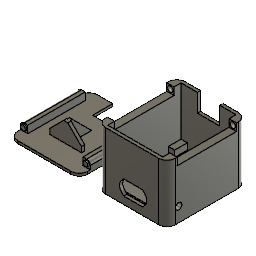
WirelessTéléInfo v8 (Autodesk Fusion 360 design; units mm, degrees)
Autodesk Fusion 360 part; units mm, degrees
form "Form1" [no effect]
sketch "Bases" plane through (0, 0, 0) normal (0, 1, 0) x (1, 0, 0)
  line L0 (7.8348, 4.1595) -> (32.8348, 4.1595)
  line L1 (36.8348, 8.1595) -> (36.8348, 37.7595)
  line L2 (32.8348, 41.7595) -> (7.8348, 41.7595)
  line L3 (3.8348, 37.7595) -> (3.8348, 8.1595)
  arc A0 (7.8348, 41.7595) -> (3.8348, 37.7595) centre (7.8348, 37.7595) ccw
  arc A1 (36.8348, 37.7595) -> (32.8348, 41.7595) centre (32.8348, 37.7595) ccw
  arc A2 (32.8348, 4.1595) -> (36.8348, 8.1595) centre (32.8348, 8.1595) ccw
  arc A3 (3.8348, 8.1595) -> (7.8348, 4.1595) centre (7.8348, 8.1595) ccw
  arc A4 (3.8348, 8.1595) -> (7.8348, 4.1595) centre (7.8348, 8.1595) ccw
  arc A5 (32.8348, 4.1595) -> (36.8348, 8.1595) centre (32.8348, 8.1595) ccw
  line L4 (3.8348, 37.7595) -> (3.8348, 8.1595)
  line L5 (36.8348, 8.1595) -> (36.8348, 37.7595)
  line L6 (7.8348, 4.1595) -> (32.8348, 4.1595)
  arc A6 (7.8348, 41.7595) -> (3.8348, 37.7595) centre (7.8348, 37.7595) ccw
  line L7 (32.8348, 41.7595) -> (7.8348, 41.7595)
  arc A7 (36.8348, 37.7595) -> (32.8348, 41.7595) centre (32.8348, 37.7595) ccw
  line L8 (-37.5541, 37.6977) -> (-37.5541, 8.0977)
  arc A8 (-8.5541, 4.0977) -> (-4.5541, 8.0977) centre (-8.5541, 8.0977) ccw
  line L9 (-33.5541, 4.0977) -> (-8.5541, 4.0977)
  line L10 (-8.5541, 41.6977) -> (-33.5541, 41.6977)
  arc A9 (-33.5541, 41.6977) -> (-37.5541, 37.6977) centre (-33.5541, 37.6977) ccw
  arc A10 (-4.5541, 37.6977) -> (-8.5541, 41.6977) centre (-8.5541, 37.6977) ccw
  arc A11 (-37.5541, 8.0977) -> (-33.5541, 4.0977) centre (-33.5541, 8.0977) ccw
  line L11 (-4.5541, 8.0977) -> (-4.5541, 37.6977)
  line L12 (-37.5541, 36.4977) -> (-34.0541, 36.4977)
  line L13 (-34.0541, 36.4977) -> (-34.0541, 9.2977)
  line L14 (-34.0541, 9.2977) -> (-37.5541, 9.2977)
  line L15 (-37.5541, 9.2977) -> (-37.5541, 36.4977)
  line L16 (-4.5541, 36.4977) -> (-8.0541, 36.4977)
  line L17 (-8.0541, 36.4977) -> (-8.0541, 9.2977)
  line L18 (-8.0541, 9.2977) -> (-4.5541, 9.2977)
  line L19 (-4.5541, 9.2977) -> (-4.5541, 36.4977)
  dimension "d14" = 4
  dimension "d15" = 4
  dimension "d16" = 37.6
  dimension "d18" = 33
  dimension "d31" = 4
  dimension "d32" = 4
  dimension "d33" = 37.6
  dimension "d34" = 33
  dimension "d35" = 4
  dimension "d36" = 4
  dimension "d37" = 37.6
  dimension "d38" = 33
  dimension "d45" = 27.2
  dimension "d46" = 3.5
  dimension "d47" = 3.5
  measures "d14" radius of A0
  measures "d15" radius of A1
  measures "d16" distance of L0 L2
  measures "d18" distance of L1 L3
  measures "d31" radius of A6
  measures "d32" radius of A7
  measures "d33" distance of L6 L7
  measures "d34" distance of L4 L5
  measures "d35" radius of A9
  measures "d36" radius of A10
  measures "d37" distance of L9 L10
  measures "d38" distance of L8 L11
  measures "d45" distance of origin
extrude "Extrude1" add sketch "Bases" along normal blind 27.25 contours L0 L1 L2 L3 A0 A1 A2 A3 A4 A5 L4 L5 L6 A6 L7 A7 makes body 1
sketch "TopBox" plane through (0, 27.25, 0) normal (0, 1, 0) x (-1, 0, 0)
  arc A0 (-3.8348, -8.1595) -> (-7.8348, -4.1595) centre (-7.8348, -8.1595) ccw
  line L0 (-7.8348, -4.1595) -> (-32.8348, -4.1595)
  arc A1 (-32.8348, -4.1595) -> (-36.8348, -8.1595) centre (-32.8348, -8.1595) ccw
  line L1 (-36.8348, -8.1595) -> (-36.8348, -37.7595)
  arc A2 (-36.8348, -37.7595) -> (-32.8348, -41.7595) centre (-32.8348, -37.7595) ccw
  line L2 (-32.8348, -41.7595) -> (-7.8348, -41.7595)
  arc A3 (-7.8348, -41.7595) -> (-3.8348, -37.7595) centre (-7.8348, -37.7595) ccw
  line L3 (-3.8348, -37.7595) -> (-3.8348, -8.1595)
  line L4 (-7.3348, -5.6595) -> (-33.3348, -5.6595)
  line L5 (-33.3348, -5.6595) -> (-33.3348, -40.2595)
  line L6 (-33.3348, -40.2595) -> (-7.3348, -40.2595)
  line L7 (-7.3348, -40.2595) -> (-7.3348, -5.6595)
  line L8 (-3.8348, -36.9595) -> (-7.3348, -36.9595)
  line L9 (-7.3348, -36.9595) -> (-7.3348, -8.9595)
  line L10 (-7.3348, -8.9595) -> (-3.8348, -8.9595)
  line L11 (-3.8348, -8.9595) -> (-3.8348, -36.9595)
  line L12 (-33.3348, -36.9595) -> (-36.8348, -36.9595)
  line L13 (-36.8348, -36.9595) -> (-36.8348, -8.9595)
  line L14 (-36.8348, -8.9595) -> (-33.3348, -8.9595)
  line L15 (-33.3348, -8.9595) -> (-33.3348, -36.9595)
  dimension "d22" = 34.6
  dimension "d23" = 26
  dimension "d24" = 1.5
  dimension "d25" = 3.5
  dimension "d28" = 28
  measures "d24" distance of L0 L4
  measures "d25" distance of L3 L7
extrude "Extrude2" cut sketch "TopBox" against normal blind 26 contours L4 L5 L6 L7 L9 L15 bodies 1
extrude "Extrude3" cut sketch "TopBox" against normal blind 3.5 contours L3 L7 L8 L9 L10 L11 | L1 L5 L12 L13 L14 L15 bodies 1
extrude "Extrude4" add sketch "Bases" along normal blind 1.25 separate body contours L8 A8 L9 L10 A9 A10 A11 L11 L12 L13 L14 L16 L17 L18 | L8 L12 L13 L14 L15 | L11 L16 L17 L18 L19 makes body 2
extrude "Extrude5" add sketch "Bases" along normal blind 4.75 contours L8 L12 L13 L14 L15 | L11 L16 L17 L18 L19 bodies 2
fillet "Fillet1" radius 1.75 1 edges at (-4.5541, 4.75, -22.8977) on bodies 2
fillet "Fillet1" radius 1.75 1 edges at (-37.5541, 4.75, -22.8977) on bodies 2
sphere "SpherePrimitive8" cut diameter 2.5 placed x (1, 0, 0) y (0, 1, 0) z (0, 0, 1) at (35.0848, 25.5, -36.9595) bodies 1
pattern_linear "R-Pattern1" count 2 spacing 28 along (0, 0, 1) count 2 spacing 29.5 along (-1, 0, 0) of "SpherePrimitive8"
sphere "SpherePrimitive9" add diameter 2.5 placed x (-1, 0, 0) y (0, 1, 0) z (0, 0, -1) at (-6.3041, 3, -36.4977) bodies 2
pattern_linear "R-Pattern2" count 2 spacing 27.2 along (0, 0, 1) count 2 spacing 29.5 along (-1, 0, 0) of "SpherePrimitive9"
sketch "CutSpheres" plane through (0, 1.25, 0) normal (0, 1, 0) x (-1, 0, 0)
  line L0 (8.0541, -36.4977) -> (4.5541, -36.4977)
  line L1 (4.5541, -36.4977) -> (4.5541, -37.6977)
  arc A0 (4.5541, -37.6977) -> (8.5541, -41.6977) centre (8.5541, -37.6977) ccw
  line L2 (8.5541, -41.6977) -> (33.5541, -41.6977)
  arc A1 (33.5541, -41.6977) -> (37.5541, -37.6977) centre (33.5541, -37.6977) ccw
  line L3 (37.5541, -37.6977) -> (37.5541, -36.4977)
  line L4 (37.5541, -36.4977) -> (34.0541, -36.4977)
  line L5 (34.0541, -36.4977) -> (34.0541, -9.2977)
  line L6 (34.0541, -9.2977) -> (37.5541, -9.2977)
  line L7 (37.5541, -9.2977) -> (37.5541, -8.0977)
  arc A2 (37.5541, -8.0977) -> (33.5541, -4.0977) centre (33.5541, -8.0977) ccw
  line L8 (33.5541, -4.0977) -> (8.5541, -4.0977)
  arc A3 (8.5541, -4.0977) -> (4.5541, -8.0977) centre (8.5541, -8.0977) ccw
  line L9 (4.5541, -8.0977) -> (4.5541, -9.2977)
  line L10 (4.5541, -9.2977) -> (8.0541, -9.2977)
  line L11 (8.0541, -9.2977) -> (8.0541, -36.4977)
  line L12 (7.5541, -37.7477) -> (5.0541, -37.7477)
  line L13 (5.0541, -37.7477) -> (5.0541, -37.0477)
  line L14 (5.0541, -37.0477) -> (7.5541, -37.0477)
  line L15 (7.5541, -37.0477) -> (7.5541, -37.7477)
  line L16 (4.5541, -8.0977) -> (4.5541, -37.6977)
  line L17 (4.5541, -36.4977) -> (8.0541, -36.4977)
  line L18 (7.5541, -8.7477) -> (5.0541, -8.7477)
  line L19 (5.0541, -8.7477) -> (5.0541, -8.0477)
  line L20 (5.0541, -8.0477) -> (7.5541, -8.0477)
  line L21 (7.5541, -8.0477) -> (7.5541, -8.7477)
  line L22 (37.0541, -8.7477) -> (34.5541, -8.7477)
  line L23 (34.5541, -8.7477) -> (34.5541, -8.0477)
  line L24 (34.5541, -8.0477) -> (37.0541, -8.0477)
  line L25 (37.0541, -8.0477) -> (37.0541, -8.7477)
  line L26 (37.0541, -37.7477) -> (34.5541, -37.7477)
  line L27 (34.5541, -37.7477) -> (34.5541, -37.0477)
  line L28 (34.5541, -37.0477) -> (37.0541, -37.0477)
  line L29 (37.0541, -37.0477) -> (37.0541, -37.7477)
  line L30 (8.0541, -9.2977) -> (4.5541, -9.2977)
  line L31 (34.0541, -9.2977) -> (37.5541, -9.2977)
  line L32 (37.5541, -36.4977) -> (34.0541, -36.4977)
  line L33 (37.5541, -37.6977) -> (37.5541, -8.0977)
  dimension "d71" = 0.5
  dimension "d72" = 2.5
  dimension "d73" = 0.55
  dimension "d74" = 0.7
  dimension "d77" = 0.55
  dimension "d78" = 0.55
  dimension "d79" = 0.55
  dimension "d80" = 0.7
  dimension "d81" = 0.7
  dimension "d82" = 0.7
  dimension "d83" = 0.5
  dimension "d84" = 0.5
  dimension "d85" = 0.5
  dimension "d86" = 2.5
  dimension "d87" = 2.5
  dimension "d88" = 2.5
  measures "d71" distance of L13 L16
  measures "d73" distance of L14 L17
  measures "d77" distance of L18 L30
  measures "d78" distance of L22 L31
  measures "d79" distance of L28 L32
  measures "d83" distance of L16 L19
  measures "d84" distance of L25 L33
  measures "d85" distance of L29 L33
extrude "Extrude6" cut sketch "CutSpheres" along normal blind 3 contours L12 L13 L14 L15 | L18 L19 L20 L21 | L22 L23 L24 L25 | L26 L27 L28 L29 bodies 2
sketch "Supports" plane through (0, 1.25, 0) normal (0, 1, 0) x (-1, 0, 0)
  line L0 (-7.3348, -40.2595) -> (-7.3348, -5.6595)
  line L1 (-7.3348, -5.6595) -> (-33.3348, -5.6595)
  line L2 (-33.3348, -5.6595) -> (-33.3348, -40.2595)
  line L3 (-33.3348, -40.2595) -> (-7.3348, -40.2595)
  line L4 (-7.3348, -5.6595) -> (-29.3348, -5.6595)
  line L5 (-29.3348, -5.6595) -> (-29.3348, -11.6595)
  line L6 (-29.3348, -11.6595) -> (-7.3348, -11.6595)
  line L7 (-7.3348, -11.6595) -> (-7.3348, -5.6595)
  line L8 (-7.3348, -40.2595) -> (-10.3348, -40.2595)
  line L9 (-10.3348, -40.2595) -> (-10.3348, -34.2595)
  line L10 (-10.3348, -34.2595) -> (-7.3348, -34.2595)
  line L11 (-7.3348, -34.2595) -> (-7.3348, -40.2595)
  line L12 (-33.3348, -40.2595) -> (-30.3348, -40.2595)
  line L13 (-30.3348, -40.2595) -> (-30.3348, -34.2595)
  line L14 (-30.3348, -34.2595) -> (-33.3348, -34.2595)
  line L15 (-33.3348, -34.2595) -> (-33.3348, -40.2595)
  dimension "d93" = 6
  dimension "d94" = 22
  dimension "d95" = 6
  dimension "d96" = 6
  dimension "d97" = 3
  dimension "d98" = 3
extrude "Extrude7" add sketch "Supports" along normal blind 3 contours L0 L3 L8 L9 L10 L11 | L0 L1 L4 L5 L6 L7 | L2 L3 L12 L13 L14 L15 bodies 1
sketch "ResetHole" plane through (36.8348, 0, 0) normal (1, 0, 0) x (0, 0, -1)
  line L0 (8.9595, 23.75) -> (8.9595, 27.25)
  line L1 (8.1595, 27.25) -> (8.1595, 0)
  line L2 (8.1595, 0) -> (37.7595, 0)
  line L3 (37.7595, 0) -> (37.7595, 27.25)
  line L4 (36.9595, 27.25) -> (36.9595, 23.75)
  line L5 (36.9595, 23.75) -> (8.9595, 23.75)
  circle A0 centre (9.6595, 6.85) radius 1.5
  line L6 (8.1595, 0) -> (37.7595, 0)
  line L7 (8.9595, 27.25) -> (8.1595, 27.25)
  line L8 (37.7595, 27.25) -> (36.9595, 27.25)
  dimension "d101" = 1.5
  dimension "d102" = 3
  dimension "d103" = 6.85
  measures "d101" distance of L1
  measures "d102" diameter of A0
  measures "d103" distance of L6
extrude "Extrude8" cut sketch "ResetHole" against normal blind 3.5 contours A0 bodies 1
sketch "USBHole" plane through (0, 0, -4.1595) normal (0, 0, 1) x (1, 0, 0)
  line L0 (7.8348, 0) -> (32.8348, 0)
  line L1 (32.8348, 0) -> (32.8348, 27.25)
  line L2 (32.8348, 27.25) -> (7.8348, 27.25)
  line L3 (7.8348, 27.25) -> (7.8348, 0)
  line L4 (16.3348, 10.55) -> (25.3348, 10.55)
  line L5 (25.3348, 3.55) -> (16.3348, 3.55)
  spline S0 degree 5 poles (16.3348, 10.55) (16.188, 10.41) (15.907, 10.13) (15.5241, 9.71) (15.0918, 9.15) (14.6906, 8.45) (14.4412, 7.75) (14.3558, 7.05) (14.4412, 6.35) (14.6906, 5.65) (15.0918, 4.95) (15.5241, 4.39) (15.907, 3.97) (16.188, 3.69) (16.3348, 3.55) knots 0 0 0 0 0 0 0.1 0.2 0.3 0.4 0.5 0.6 0.7 0.8 0.9 1 1 1 1 1 1
  spline S1 degree 5 poles (25.3348, 3.55) (25.4817, 3.69) (25.7626, 3.97) (26.1456, 4.39) (26.5779, 4.95) (26.979, 5.65) (27.2285, 6.35) (27.3139, 7.05) (27.2285, 7.75) (26.979, 8.45) (26.5779, 9.15) (26.1456, 9.71) (25.7626, 10.13) (25.4817, 10.41) (25.3348, 10.55) knots 0 0 0 0 0 0 0.1 0.2 0.3 0.4 0.5 0.6 0.7 0.8 0.9 1 1 1 1 1 1
  line L6 (16.3348, 10.55) -> (16.3348, 3.55)
  line L7 (25.3348, 10.55) -> (25.3348, 3.55)
  line L8 (7.8348, 3.55) -> (32.8348, 3.55)
  line L9 (7.8348, 0) -> (32.8348, 0)
  dimension "d104" = 9
  dimension "d105" = 7
  dimension "d106" = 4
  dimension "d107" = 4
  dimension "d108" = 4
  dimension "d109" = 4
  dimension "d115" = 7.05
  dimension "d138" = 4
  measures "d115" distance of L9
extrude "Extrude9" cut sketch "USBHole" against normal blind 1.5 contours L4 L5 L6 L7 L8 | S0 L6 | S1 L7 bodies 1
sketch "BornierHole" plane through (0, 0, -41.7595) normal (0, 0, -1) x (-1, 0, 0)
  line L0 (-32.8348, 0) -> (-7.8348, 0)
  line L1 (-7.8348, 0) -> (-7.8348, 27.25)
  line L2 (-7.8348, 27.25) -> (-32.8348, 27.25)
  line L3 (-32.8348, 27.25) -> (-32.8348, 0)
  line L4 (-25.5848, 27.25) -> (-15.0848, 27.25)
  line L5 (-15.0848, 27.25) -> (-15.0848, 18.75)
  line L6 (-15.0848, 18.75) -> (-25.5848, 18.75)
  line L7 (-25.5848, 18.75) -> (-25.5848, 27.25)
  dimension "d116" = 10.5
  dimension "d117" = 8.5
  measures "d116" distance of origin
  measures "d117" distance of origin
extrude "Extrude10" cut sketch "BornierHole" against normal blind 1.5 contours L2 L4 L5 L6 L7 bodies 1
sketch "BordnierHoleAndMaintainLeg" plane through (0, 1.25, 0) normal (0, 1, 0) x (-1, 0, 0)
  line L0 (8.0541, -36.4977) -> (4.5541, -36.4977)
  line L1 (4.5541, -36.4977) -> (4.5541, -37.6977)
  arc A0 (4.5541, -37.6977) -> (8.5541, -41.6977) centre (8.5541, -37.6977) ccw
  line L2 (8.5541, -41.6977) -> (33.5541, -41.6977)
  arc A1 (33.5541, -41.6977) -> (37.5541, -37.6977) centre (33.5541, -37.6977) ccw
  line L3 (37.5541, -37.6977) -> (37.5541, -36.4977)
  line L4 (37.5541, -36.4977) -> (34.0541, -36.4977)
  line L5 (34.0541, -36.4977) -> (34.0541, -9.2977)
  line L6 (34.0541, -9.2977) -> (37.5541, -9.2977)
  line L7 (37.5541, -9.2977) -> (37.5541, -8.0977)
  arc A2 (37.5541, -8.0977) -> (33.5541, -4.0977) centre (33.5541, -8.0977) ccw
  line L8 (33.5541, -4.0977) -> (8.5541, -4.0977)
  arc A3 (8.5541, -4.0977) -> (4.5541, -8.0977) centre (8.5541, -8.0977) ccw
  line L9 (4.5541, -8.0977) -> (4.5541, -9.2977)
  line L10 (4.5541, -9.2977) -> (8.0541, -9.2977)
  line L11 (8.0541, -9.2977) -> (8.0541, -36.4977)
  line L12 (26.3041, -41.6977) -> (15.8041, -41.6977)
  line L13 (15.8041, -41.6977) -> (15.8041, -32.1977)
  line L14 (15.8041, -32.1977) -> (26.3041, -32.1977)
  line L15 (26.3041, -32.1977) -> (26.3041, -41.6977)
  line L16 (28.5541, -14.1977) -> (13.5541, -14.1977)
  line L17 (13.5541, -14.1977) -> (13.5541, -15.6977)
  line L18 (13.5541, -15.6977) -> (28.5541, -15.6977)
  line L19 (28.5541, -15.6977) -> (28.5541, -14.1977)
  line L20 (21.8041, -15.6977) -> (20.3041, -15.6977)
  line L21 (20.3041, -15.6977) -> (20.3041, -25.6977)
  line L22 (20.3041, -25.6977) -> (21.8041, -25.6977)
  line L23 (21.8041, -25.6977) -> (21.8041, -15.6977)
  line L24 (34.0541, -14.1977) -> (8.0541, -14.1977)
  dimension "d120" = 10.5
  dimension "d121" = 9.5
  dimension "d122" = 1.5
  dimension "d123" = 1.5
  dimension "d124" = 15
  dimension "d125" = 10
  dimension "d126" = 27.5
  measures "d120" distance of origin
  measures "d122" distance of L16 L18
  measures "d123" distance of L21 L23
  measures "d125" distance of origin
  measures "d126" distance of L2 L24
extrude "Extrude11" cut sketch "BordnierHoleAndMaintainLeg" against normal blind 1.25 contours L2 L12 L13 L14 L15 bodies 2
extrude "Extrude12" add sketch "BordnierHoleAndMaintainLeg" along normal blind 9 contours L16 L17 L18 L19 L20 L24 | L18 L20 L21 L22 L23 bodies 2
chamfer "Chamfer1" distance 6.5 angle 45 2 edges at (-28.5541, 10.25, -14.9477) (-13.5541, 10.25, -14.9477) on bodies 2
chamfer "Chamfer2" distance 9 angle 45 1 edges at (-21.0541, 10.25, -25.6977) on bodies 2
sketch "ModuleName" plane through (0, 0, 0) normal (0, -1, 0) x (1, 0, 0)
  line L0 (-26.3041, -41.6977) -> (-26.3041, -32.1977)
  line L1 (-26.3041, -32.1977) -> (-15.8041, -32.1977)
  line L2 (-15.8041, -32.1977) -> (-15.8041, -41.6977)
  line L3 (-15.8041, -41.6977) -> (-8.5541, -41.6977)
  arc A0 (-8.5541, -41.6977) -> (-4.5541, -37.6977) centre (-8.5541, -37.6977) ccw
  line L4 (-4.5541, -37.6977) -> (-4.5541, -8.0977)
  arc A1 (-4.5541, -8.0977) -> (-8.5541, -4.0977) centre (-8.5541, -8.0977) ccw
  line L5 (-8.5541, -4.0977) -> (-33.5541, -4.0977)
  arc A2 (-33.5541, -4.0977) -> (-37.5541, -8.0977) centre (-33.5541, -8.0977) ccw
  line L6 (-37.5541, -8.0977) -> (-37.5541, -37.6977)
  arc A3 (-37.5541, -37.6977) -> (-33.5541, -41.6977) centre (-33.5541, -37.6977) ccw
  line L7 (-33.5541, -41.6977) -> (-26.3041, -41.6977)
  line L8 (-8.3337, -24.7187) -> (-33.0602, -24.7187) construction
  line L9 (-33.0602, -24.7187) -> (-33.0602, -29.7187) construction
  line L10 (-33.0602, -29.7187) -> (-8.3337, -29.7187) construction
  line L11 (-8.3337, -29.7187) -> (-8.3337, -24.7187) construction
  line L12 (-10.3438, -18.9177) -> (-30.6074, -18.9177) construction
  line L13 (-30.6074, -18.9177) -> (-30.6074, -23.9177) construction
  line L14 (-30.6074, -23.9177) -> (-10.3438, -23.9177) construction
  line L15 (-10.3438, -23.9177) -> (-10.3438, -18.9177) construction
  line L16 (-10.9219, -13.5277) -> (-29.8037, -13.5277) construction
  line L17 (-29.8037, -13.5277) -> (-29.8037, -18.5277) construction
  line L18 (-29.8037, -18.5277) -> (-10.9219, -18.5277) construction
  line L19 (-10.9219, -18.5277) -> (-10.9219, -13.5277) construction
  line L20 (-15.3778, -7.1463) -> (-24.8529, -7.1463) construction
  line L21 (-24.8529, -7.1463) -> (-24.8529, -12.1463) construction
  line L22 (-24.8529, -12.1463) -> (-15.3778, -12.1463) construction
  line L23 (-15.3778, -12.1463) -> (-15.3778, -7.1463) construction
  text T0 "DomoChip" font "Arial" height 5 bold align ink ink in box 0 x 0 at (-8.3337, -24.7187) x (-1, 0) y (0, -1) spacing 1 kerned height is em
  text T1 "Wireless" font "Arial" height 5 bold align ink ink in box 0 x 0 at (-10.3438, -18.9177) x (-1, 0) y (0, -1) spacing 1 kerned height is em
  text T2 "TéléInfo" font "Arial" height 5 bold align ink ink in box 0 x 0 at (-10.9219, -13.5277) x (-1, 0) y (0, -1) spacing 1 kerned height is em
  text T3 "V2.1" font "Arial" height 5 bold align ink ink in box 0 x 0 at (-15.3778, -7.1463) x (-1, 0) y (0, -1) spacing 1 kerned height is em
extrude "Extrude13" cut sketch "ModuleName" against normal blind 0.5 text T0 T1 T2 T3 bodies 2
equation "_width = 34.6 mm" comment "width of the box (affects the length of the hinges)"
equation "_length = 26 mm" comment "length of the box"
equation "_height = 26 mm" comment "height of the box"
equation "_rounding = 4 mm" comment "rounding radius of the corners of the box"
equation "_minimumWallThickness = 0.5 mm" comment "thickness of the walls around the magnets"
equation "_sidewallThickness = 1.5 mm" comment "thickness of the side walls without the hinge"
equation "_horizontalThickness = 1.25 mm" comment "thickness of the bottom of the box or the top of the lid"
equation "_magnetDiameter = 2.5 mm" comment "diameter of magnets in the hinge"
equation "_magnetHeight = 1 mm" comment "height magnets in the hinge"
equation "_hingeGap = 0.4 mm" comment "gap bewteen the lid and box parts"
equation "_hingeOverlap = 0.15 mm" comment "Size of lid's spheres that go into box holes"
equation "d14 = _rounding"
equation "d15 = _rounding"
equation "d16 = _width + 2 * _sidewallThickness"
equation "d18 = _length + 4 * _minimumWallThickness + 2 * _magnetDiameter"
equation "d20 = _height + _horizontalThickness"
equation "d22 = _width"
equation "d23 = _length"
equation "d24 = _sidewallThickness"
equation "d25 = 2 * _minimumWallThickness + _magnetDiameter"
equation "d26 = -_height"
equation "d28 = _width + 2 * _sidewallThickness - 2 * _rounding - 2 * _magnetHeight + _hingeGap"
equation "d29 = -_magnetDiameter - 2 * _minimumWallThickness"
equation "d31 = _rounding"
equation "d32 = _rounding"
equation "d33 = _width + 2 * _sidewallThickness"
equation "d34 = _length + 4 * _minimumWallThickness + 2 * _magnetDiameter"
equation "d35 = _rounding"
equation "d36 = _rounding"
equation "d37 = _width + 2 * _sidewallThickness"
equation "d38 = _length + 4 * _minimumWallThickness + 2 * _magnetDiameter"
equation "d43 = _horizontalThickness"
equation "d45 = _width + 2 * _sidewallThickness - 2 * _rounding - 2 * _magnetHeight - _hingeGap"
equation "d46 = _magnetDiameter + 2 * _minimumWallThickness"
equation "d47 = _magnetDiameter + 2 * _minimumWallThickness"
equation "d48 = _horizontalThickness + _magnetDiameter + 2 * _minimumWallThickness"
equation "d50 = ( _magnetDiameter + 2 * _minimumWallThickness ) / 2"
equation "d51 = ( _magnetDiameter + 2 * _minimumWallThickness ) / 2"
equation "d59 = _width + 2 * _sidewallThickness - 2 * _rounding - 2 * _magnetHeight + _hingeGap"
equation "d60 = -_length - _magnetDiameter - 2 * _minimumWallThickness"
equation "d64 = _width + 2 * _sidewallThickness - 2 * _rounding - 2 * _magnetHeight - _hingeGap"
equation "d65 = -_length - _magnetDiameter - 2 * _minimumWallThickness"
equation "d71 = _minimumWallThickness"
equation "d72 = _magnetDiameter"
equation "d73 = _hingeGap + _hingeOverlap"
equation "d74 = _magnetDiameter / 2 - _hingeGap - _hingeOverlap"
equation "d75 = _minimumWallThickness + _magnetDiameter"
equation "d77 = _hingeGap + _hingeOverlap"
equation "d78 = _hingeGap + _hingeOverlap"
equation "d79 = _hingeGap + _hingeOverlap"
equation "d80 = _magnetDiameter / 2 - _hingeGap - _hingeOverlap"
equation "d81 = _magnetDiameter / 2 - _hingeGap - _hingeOverlap"
equation "d82 = _magnetDiameter / 2 - _hingeGap - _hingeOverlap"
equation "d83 = _minimumWallThickness"
equation "d84 = _minimumWallThickness"
equation "d85 = _minimumWallThickness"
equation "d86 = _magnetDiameter"
equation "d87 = _magnetDiameter"
equation "d88 = _magnetDiameter"
equation "d101 = 4 mm - _rounding + _sidewallThickness"
equation "d103 = _horizontalThickness + 3 mm + 1.6 mm + 1 mm"
equation "d111 = -_magnetDiameter - 2 * _minimumWallThickness"
equation "d113 = -_sidewallThickness"
equation "d115 = 3 mm + 2.8 mm + _horizontalThickness"
equation "d118 = -_sidewallThickness"
equation "d121 = 8 mm + _sidewallThickness"
equation "d126 = 26 mm + _sidewallThickness"
equation "d127 = -_horizontalThickness"
equation "d136 = _magnetDiameter"
equation "d137 = _magnetDiameter"
named bodies: "WirelessTeleInfo Box", "WirelessTeleInfo Lid"
